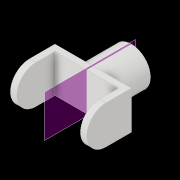
# Autodesk Inventor part: L1_0.1
Saved by Autodesk Inventor 2019 (Build 230136000, 136)
## iProperties
Created: 2021-08-06
Part Number: L1_0.1
Material: ABS 플라스틱
Document SubType Name: Modeling
Designer: YoonJunHeon
Density: 1.06 g/cm^3
Appearance: 매끄러움 - 흰색
Mass: 40534.4 g
Surface Area: 11012.4 cm^2
Volume: 38240 cm^3
Author: YoonJunHeon
Autodesk Inventor part; units mm, degrees
ref_plane "YZ Plane" through (0, 0, 0) normal (1, 0, 0) x (0, 1, 0)
ref_plane "XZ Plane" through (0, 0, 0) normal (0, 1, 0) x (-1, 0, 0)
ref_plane "XY Plane" through (0, 0, 0) normal (0, 0, 1) x (1, 0, 0)
sketch "스케치1" plane through (0, 0, 0) normal (0, 0, 1) x (1, 0, 0)
  circle A0 centre (0, 0) radius 15
  dimension "d0" = 30
  constraints: 1 centre point, 1 coincident
  measures "d0" diameter of A0
extrude "돌출1" add sketch "스케치1" along normal blind 30
sketch "스케치2" plane through (0, 0, 30) normal (0, 0, 1) x (1, 0, 0)
  line L0 (30, 15) -> (-30, 15)
  line L1 (-30, 15) -> (-30, -15)
  line L2 (-30, -15) -> (30, -15)
  line L3 (30, -15) -> (30, 15)
  line L4 (30, 15) -> (-30, -15) construction
  line L5 (-30, 15) -> (30, -15) construction
  point P0 (0, 0)
  dimension "d3" = 60
  dimension "d4" = 30
  constraints: 12 end point, 2 midpoint, 2 parallel, 1 horizontal, 1 perpendicular
  measures "d3" distance of L2.end L1.end
  measures "d4" distance of L1.end L0.end
extrude "돌출2" add sketch "스케치2" along normal blind 5
sketch "스케치3" plane through (30, -15, 30) normal (1, 0, 0) x (0, 0, -1)
  line L0 (0, 0) -> (0, 30) projected
  line L1 (0, 30) -> (-5, 30) projected
  line L2 (-5, 0) -> (-5, 30) projected
  line L3 (0, 0) -> (-5, 0) projected
  line L4 (-5, 0) -> (-20, 0)
  line L5 (-20, 30) -> (-5, 30)
  line L6 (-5, 30) -> (-5, 0)
  line L7 (0, 0) -> (-5, 0) projected
  line L8 (0, 30) -> (-5, 30) projected
  arc A0 (-20, 30) -> (-20, 0) centre (-20, 15) ccw
  point P0 (30, 15)
  dimension "d10" = 15
  dimension "d11" = 15
  dimension "d12" = 15
  constraints: 6 end point, 2 collinear, 2 point on circle, 1 centre point, 1 horizontal, 1 parallel
  measures "d10" distance of L5.start L5.end
  measures "d11" distance of L2.start L4.end
  measures "d12" radius of A0
extrude "돌출3" add sketch "스케치3" against normal blind 5 contours L4 A0 L5 L2
mirror "미러1" about plane through (0, 0, 0) normal (1, 0, 0) of "돌출3"
ref_plane "작업 평면1" through (0, 0, 0) normal (1, 0, 0) x (0, 1, 0)
